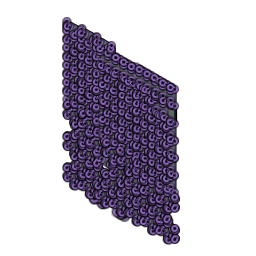
Press Fit v3 (Autodesk Fusion 360 design; units mm, degrees)
Autodesk Fusion 360 part; units mm, degrees
(part 1 of 4)
sketch "Sketch2" plane through (0, 0, 0) normal (0, 0, 1) x (1, 0, 0)
  line L0 (0, 0) -> (50.15, 0)
  line L1 (50.15, 0) -> (50.15, 50.15)
  line L2 (50.15, 50.15) -> (0, 50.15)
  line L3 (0, 50.15) -> (0, 0)
  line L4 (100.15, 0) -> (130.3, 0)
  line L5 (130.3, 0) -> (145.375, 26.1107)
  line L6 (145.375, 26.1107) -> (130.3, 52.2213)
  line L7 (130.3, 52.2213) -> (100.15, 52.2213)
  line L8 (100.15, 52.2213) -> (85.075, 26.1107)
  line L9 (85.075, 26.1107) -> (100.15, 0)
  line L10 (180.3, 50.15) -> (205.45, 50.15)
  line L11 (205.45, 50.15) -> (205.45, 0)
  line L12 (205.45, 0) -> (180.3, 0)
  line L13 (180.3, 0) -> (180.3, 50.15)
  line L14 (23.525, 50.15) -> (26.625, 50.15)
  line L15 (26.625, 50.15) -> (26.625, 40)
  line L16 (26.625, 40) -> (23.525, 40)
  line L17 (23.525, 40) -> (23.525, 50.15)
  line L18 (0, 26.625) -> (10.15, 26.625)
  line L19 (10.15, 26.625) -> (10.15, 23.525)
  line L20 (10.15, 23.525) -> (0, 23.525)
  line L21 (0, 23.525) -> (0, 26.625)
  line L22 (50.15, 26.625) -> (40, 26.625)
  line L23 (40, 26.625) -> (40, 23.525)
  line L24 (40, 23.525) -> (50.15, 23.525)
  line L25 (50.15, 23.525) -> (50.15, 26.625)
  line L26 (26.625, 0) -> (23.525, 0)
  line L27 (23.525, 0) -> (23.525, 10.15)
  line L28 (23.525, 10.15) -> (26.625, 10.15)
  line L29 (26.625, 10.15) -> (26.625, 0)
  line L30 (100.15, 52.2213) -> (130.3, 0) construction
  line L31 (130.3, 52.2213) -> (100.15, 0) construction
  line L32 (85.075, 26.1107) -> (145.375, 26.1107) construction
  line L33 (192.875, 50.15) -> (192.875, 0) construction
  line L34 (25.075, 50.15) -> (25.075, -50.15) construction
  line L35 (0, 25.075) -> (50.15, 25.075) construction
  line L36 (99.2551, 50.6713) -> (101.9398, 52.2213)
  line L37 (101.9398, 52.2213) -> (107.0148, 43.4312)
  line L38 (107.0148, 43.4312) -> (104.3301, 41.8812)
  line L39 (104.3301, 41.8812) -> (99.2551, 50.6713)
  line L40 (128.5102, 52.2213) -> (131.1949, 50.6713)
  line L41 (131.1949, 50.6713) -> (126.1199, 41.8812)
  line L42 (126.1199, 41.8812) -> (123.4352, 43.4312)
  line L43 (123.4352, 43.4312) -> (128.5102, 52.2213)
  line L44 (144.4801, 27.6607) -> (144.4801, 24.5607)
  line L45 (144.4801, 24.5607) -> (134.3301, 24.5607)
  line L46 (134.3301, 24.5607) -> (134.3301, 27.6607)
  line L47 (134.3301, 27.6607) -> (144.4801, 27.6607)
  line L48 (128.5102, 0) -> (131.1949, 1.55)
  line L49 (131.1949, 1.55) -> (126.1199, 10.3402)
  line L50 (126.1199, 10.3402) -> (123.4352, 8.7902)
  line L51 (123.4352, 8.7902) -> (128.5102, 0)
  line L52 (101.9398, 0) -> (99.2551, 1.55)
  line L53 (99.2551, 1.55) -> (104.3301, 10.3402)
  line L54 (104.3301, 10.3402) -> (107.0148, 8.7902)
  line L55 (107.0148, 8.7902) -> (101.9398, 0)
  line L56 (85.9699, 24.5607) -> (85.9699, 27.6607)
  line L57 (85.9699, 27.6607) -> (96.1199, 27.6607)
  line L58 (96.1199, 27.6607) -> (96.1199, 24.5607)
  line L59 (96.1199, 24.5607) -> (85.9699, 24.5607)
  line L60 (191.325, 0) -> (194.425, 0)
  line L61 (194.425, 0) -> (194.425, 10.15)
  line L62 (194.425, 10.15) -> (191.325, 10.15)
  line L63 (191.325, 10.15) -> (191.325, 0)
  line L64 (191.325, 50.15) -> (194.425, 50.15)
  line L65 (194.425, 50.15) -> (194.425, 40)
  line L66 (194.425, 40) -> (191.325, 40)
  line L67 (191.325, 40) -> (191.325, 50.15)
  point P0 (115.225, 26.1107)
  dimension "d5" = 3.1
  dimension "d8" = 10.15
  dimension "d9" = 30.15
  dimension "d10" = 50.15
  dimension "d12" = 25.15
  dimension "d13" = 50.15
  dimension "d14" = 50
  dimension "d15" = 50
  dimension "d20" = 50.15
  constraint horizontal L0
  constraint vertical L1
  constraint horizontal L2
  constraint vertical L3
  constraint coincident L0.start L3.end
  constraint horizontal L4
  constraint horizontal L10
  constraint vertical L11
  constraint horizontal L12
  constraint vertical L13
  constraint horizontal L14
  constraint vertical L15
  constraint horizontal L16
  constraint vertical L17
  constraint coincident L2 L14.start
  constraint horizontal L18
  constraint vertical L19
  constraint horizontal L20
  constraint vertical L21
  constraint horizontal L22
  constraint vertical L23
  constraint horizontal L24
  constraint vertical L25
  constraint coincident L1 L22.start
  constraint vertical L27
  constraint horizontal L28
  constraint vertical L29
  constraint coincident L0 L26.start
  constraint horizontal L32
  constraint midpoint L10 L33.start
  constraint midpoint L12 L33.end
  constraint midpoint L2 L34.start
  constraint midpoint L21 L35.start
  constraint midpoint L25 L35.end
  constraint vertical L34
  constraint horizontal L35
  constraint perpendicular L36 L37
  constraint parallel L36 L38
  constraint parallel L37 L39
  constraint coincident L7 L36.end
  constraint coincident L8 L36.start
  constraint perpendicular L40 L41
  constraint parallel L40 L42
  constraint parallel L41 L43
  constraint coincident L6 L40.end
  constraint coincident L7 L40.start
  constraint perpendicular L44 L45
  constraint parallel L44 L46
  constraint parallel L45 L47
  constraint coincident L5 L44.end
  constraint perpendicular L32 L44
  constraint coincident L6 L44.start
  constraint perpendicular L48 L49
  constraint parallel L48 L50
  constraint parallel L49 L51
  constraint perpendicular L30 L48
  constraint coincident L4 L48.start
  constraint perpendicular L52 L53
  constraint parallel L52 L54
  constraint parallel L53 L55
  constraint coincident L9 L52.end
  constraint coincident L4 L52.start
  constraint perpendicular L56 L57
  constraint parallel L56 L58
  constraint parallel L57 L59
  constraint coincident L8 L56.end
  constraint perpendicular L4 L56
  constraint coincident L9 L56.start
  constraint symmetric L31 L53 L55
  constraint symmetric L30 L37 L39
  constraint symmetric L31 L41 L43
  constraint symmetric L30 L49 L51
  constraint equal L16 L19
  constraint equal L16 L23
  constraint equal L23 L28
  constraint equal L28 L58
  constraint equal L38 L58
  constraint equal L38 L42
  constraint equal L42 L46
  constraint equal L46 L50
  constraint equal L50 L54
  constraint equal L39 L57
  constraint equal L39 L43
  constraint equal L43 L47
  constraint equal L47 L49
  constraint equal L49 L55
  constraint symmetric L0 L2 L35
  constraint equal L15 L59
  constraint equal L15 L20
  constraint equal L20 L24
  constraint equal L24 L29
  constraint collinear L0 L4
  constraint horizontal L60
  constraint vertical L61
  constraint horizontal L62
  constraint vertical L63
  constraint coincident L12 L60.start
  constraint horizontal L64
  constraint vertical L65
  constraint horizontal L66
  constraint vertical L67
  constraint coincident L10 L64.start
  constraint collinear L4 L12
  constraint equal L61 L65
  constraint equal L45 L65
  constraint equal L62 L66
  constraint equal L50 L62
  constraint midpoint L0 L34
  constraint collinear L3 L21
  measures "d5" distance of L18.end L19.end
  measures "d8" distance of L56.end L57.end
  measures "d9" distance of L4.start L4.end
  measures "d10" distance of L0.end L1.end
  measures "d12" distance of L11.end L12.end
  measures "d13" distance of L10.end L11.end
  measures "d14" distance of L0.end L4.start
  measures "d15" distance of L4.end L12.end
  measures "d20" distance of L0.start L0.end
extrude "Extrude1" add sketch "Sketch2" along normal blind 5 contours L0 L1 L2 L3 L15 L16 L17 L18 L19 L20 L22 L23 L24 L27 L28 L29 | L4 L5 L6 L7 L8 L9 L37 L38 L39 L41 L42 L43 L45 L46 L47 L49 L50 L51 L53 L54 L55 L57 L58 L59 | L10 L11 L12 L13 L61 L62 L63 L65 L66 L67 makes body 1 at (11.225, 38.925, 0) makes body 2 at (112.4883, 31.8842, 0) makes body 3 at (183.975, 30.05, 0)
sketch "Sketch7" plane through (0, 0, 0) normal (0, 0, -1) x (1, 0, 0)
  line L0 (50.15, -50.15) -> (50.15, -26.625)
  line L1 (50.15, -26.625) -> (40, -26.625)
  line L2 (40, -26.625) -> (40, -23.525)
  line L3 (40, -23.525) -> (50.15, -23.525)
  line L4 (50.15, -23.525) -> (50.15, 0)
  line L5 (50.15, 0) -> (26.625, 0)
  line L6 (26.625, 0) -> (26.625, -10.15)
  line L7 (26.625, -10.15) -> (23.525, -10.15)
  line L8 (23.525, -10.15) -> (23.525, 0)
  line L9 (23.525, 0) -> (0, 0)
  line L10 (0, 0) -> (0, -23.525)
  line L11 (0, -23.525) -> (10.15, -23.525)
  line L12 (10.15, -23.525) -> (10.15, -26.625)
  line L13 (10.15, -26.625) -> (0, -26.625)
  line L14 (0, -26.625) -> (0, -50.15)
  line L15 (0, -50.15) -> (23.525, -50.15)
  line L16 (23.525, -50.15) -> (23.525, -40)
  line L17 (23.525, -40) -> (26.625, -40)
  line L18 (26.625, -40) -> (26.625, -50.15)
  line L19 (26.625, -50.15) -> (50.15, -50.15)
  line L20 (144.4801, -24.5607) -> (131.1949, -1.55)
  line L21 (131.1949, -1.55) -> (126.1199, -10.3402)
  line L22 (126.1199, -10.3402) -> (123.4352, -8.7902)
  line L23 (123.4352, -8.7902) -> (128.5102, 0)
  line L24 (128.5102, 0) -> (101.9398, 0)
  line L25 (101.9398, 0) -> (107.0148, -8.7902)
  line L26 (107.0148, -8.7902) -> (104.3301, -10.3402)
  line L27 (104.3301, -10.3402) -> (99.2551, -1.55)
  line L28 (99.2551, -1.55) -> (85.9699, -24.5607)
  line L29 (85.9699, -24.5607) -> (96.1199, -24.5607)
  line L30 (96.1199, -24.5607) -> (96.1199, -27.6607)
  line L31 (96.1199, -27.6607) -> (85.9699, -27.6607)
  line L32 (85.9699, -27.6607) -> (99.2551, -50.6713)
  line L33 (99.2551, -50.6713) -> (104.3301, -41.8812)
  line L34 (104.3301, -41.8812) -> (107.0148, -43.4312)
  line L35 (107.0148, -43.4312) -> (101.9398, -52.2213)
  line L36 (101.9398, -52.2213) -> (128.5102, -52.2213)
  line L37 (128.5102, -52.2213) -> (123.4352, -43.4312)
  line L38 (123.4352, -43.4312) -> (126.1199, -41.8812)
  line L39 (126.1199, -41.8812) -> (131.1949, -50.6713)
  line L40 (131.1949, -50.6713) -> (144.4801, -27.6607)
  line L41 (144.4801, -27.6607) -> (134.3301, -27.6607)
  line L42 (134.3301, -27.6607) -> (134.3301, -24.5607)
  line L43 (134.3301, -24.5607) -> (144.4801, -24.5607)
  line L44 (194.425, -40) -> (194.425, -50.15)
  line L45 (194.425, -50.15) -> (205.45, -50.15)
  line L46 (205.45, -50.15) -> (205.45, 0)
  line L47 (205.45, 0) -> (194.425, 0)
  line L48 (194.425, 0) -> (194.425, -10.15)
  line L49 (194.425, -10.15) -> (191.325, -10.15)
  line L50 (191.325, -10.15) -> (191.325, 0)
  line L51 (191.325, 0) -> (180.3, 0)
  line L52 (180.3, 0) -> (180.3, -50.15)
  line L53 (180.3, -50.15) -> (191.325, -50.15)
  line L54 (191.325, -50.15) -> (191.325, -40)
  line L55 (191.325, -40) -> (194.425, -40)
chamfer "Chamfer1" distance 1.5 angle 45 24 edges at (101.9398, 52.2213, 2.5) (85.9699, 27.6607, 2.5) (128.5102, 52.2213, 2.5) (99.2551, 1.55, 2.5) (101.9398, 0, 2.5) (128.5102, 0, 2.5) (131.1949, 1.55, 2.5) (144.4801, 27.6607, 2.5) (131.1949, 50.6713, 2.5) (144.4801, 24.5607, 2.5) (85.9699, 24.5607, 2.5) (99.2551, 50.6713, 2.5) (23.525, 50.15, 2.5) (26.625, 50.15, 2.5) (0, 26.625, 2.5) (0, 23.525, 2.5) (26.625, 0, 2.5) (50.15, 23.525, 2.5) (23.525, 0, 2.5) (50.15, 26.625, 2.5) (191.325, 50.15, 2.5) (194.425, 50.15, 2.5) (194.425, 0, 2.5) (191.325, 0, 2.5) on bodies 1 2 3
sketch "Sketch5" plane through (0, 0, 5) normal (0, 0, 1) x (-1, 0, 0)
  line L0 (-50.15, -28.125) -> (-50.15, -50.15)
  line L1 (-50.15, -50.15) -> (-28.125, -50.15)
  line L2 (-26.625, -48.65) -> (-26.625, -40)
  line L3 (-26.625, -40) -> (-23.525, -40)
  line L4 (-23.525, -40) -> (-23.525, -48.65)
  line L5 (-22.025, -50.15) -> (0, -50.15)
  line L6 (0, -50.15) -> (0, -28.125)
  line L7 (-1.5, -26.625) -> (-10.15, -26.625)
  line L8 (-10.15, -26.625) -> (-10.15, -23.525)
  line L9 (-10.15, -23.525) -> (-1.5, -23.525)
  line L10 (0, -22.025) -> (0, 0)
  line L11 (0, 0) -> (-22.025, 0)
  line L12 (-23.525, -1.5) -> (-23.525, -10.15)
  line L13 (-23.525, -10.15) -> (-26.625, -10.15)
  line L14 (-26.625, -10.15) -> (-26.625, -1.5)
  line L15 (-28.125, 0) -> (-50.15, 0)
  line L16 (-50.15, 0) -> (-50.15, -22.025)
  line L17 (-48.65, -23.525) -> (-40, -23.525)
  line L18 (-40, -23.525) -> (-40, -26.625)
  line L19 (-40, -26.625) -> (-48.65, -26.625)
  line L20 (-131.9449, -2.849) -> (-143.7301, -23.2616)
  line L21 (-142.9801, -24.5607) -> (-134.3301, -24.5607)
  line L22 (-134.3301, -24.5607) -> (-134.3301, -27.6607)
  line L23 (-134.3301, -27.6607) -> (-142.9801, -27.6607)
  line L24 (-143.7301, -28.9597) -> (-131.9449, -49.3723)
  line L25 (-130.4449, -49.3723) -> (-126.1199, -41.8812)
  line L26 (-126.1199, -41.8812) -> (-123.4352, -43.4312)
  line L27 (-123.4352, -43.4312) -> (-127.7602, -50.9223)
  line L28 (-127.0102, -52.2213) -> (-103.4398, -52.2213)
  line L29 (-102.6898, -50.9223) -> (-107.0148, -43.4312)
  line L30 (-107.0148, -43.4312) -> (-104.3301, -41.8812)
  line L31 (-104.3301, -41.8812) -> (-100.0051, -49.3723)
  line L32 (-98.5051, -49.3723) -> (-86.7199, -28.9597)
  line L33 (-87.4699, -27.6607) -> (-96.1199, -27.6607)
  line L34 (-96.1199, -27.6607) -> (-96.1199, -24.5607)
  line L35 (-96.1199, -24.5607) -> (-87.4699, -24.5607)
  line L36 (-86.7199, -23.2616) -> (-98.5051, -2.849)
  line L37 (-100.0051, -2.849) -> (-104.3301, -10.3402)
  line L38 (-104.3301, -10.3402) -> (-107.0148, -8.7902)
  line L39 (-107.0148, -8.7902) -> (-102.6898, -1.299)
  line L40 (-103.4398, 0) -> (-127.0102, 0)
  line L41 (-127.7602, -1.299) -> (-123.4352, -8.7902)
  line L42 (-123.4352, -8.7902) -> (-126.1199, -10.3402)
  line L43 (-126.1199, -10.3402) -> (-130.4449, -2.849)
  line L44 (-194.425, -48.65) -> (-194.425, -40)
  line L45 (-194.425, -40) -> (-191.325, -40)
  line L46 (-191.325, -40) -> (-191.325, -48.65)
  line L47 (-189.825, -50.15) -> (-180.3, -50.15)
  line L48 (-180.3, -50.15) -> (-180.3, 0)
  line L49 (-180.3, 0) -> (-189.825, 0)
  line L50 (-191.325, -1.5) -> (-191.325, -10.15)
  line L51 (-191.325, -10.15) -> (-194.425, -10.15)
  line L52 (-194.425, -10.15) -> (-194.425, -1.5)
  line L53 (-195.925, 0) -> (-205.45, 0)
  line L54 (-205.45, 0) -> (-205.45, -50.15)
  line L55 (-205.45, -50.15) -> (-195.925, -50.15)
  line L56 (-48.65, -26.625) -> (-50.15, -28.125)
  line L57 (-28.125, -50.15) -> (-26.625, -48.65)
  line L58 (-23.525, -48.65) -> (-22.025, -50.15)
  line L59 (0, -28.125) -> (-1.5, -26.625)
  line L60 (-1.5, -23.525) -> (0, -22.025)
  line L61 (-22.025, 0) -> (-23.525, -1.5)
  line L62 (-26.625, -1.5) -> (-28.125, 0)
  line L63 (-50.15, -22.025) -> (-48.65, -23.525)
  line L64 (-100.0051, -49.3723) -> (-98.5051, -49.3723)
  line L65 (-86.7199, -28.9597) -> (-87.4699, -27.6607)
  line L66 (-87.4699, -24.5607) -> (-86.7199, -23.2616)
  line L67 (-98.5051, -2.849) -> (-100.0051, -2.849)
  line L68 (-102.6898, -1.299) -> (-103.4398, 0)
  line L69 (-127.0102, 0) -> (-127.7602, -1.299)
  line L70 (-130.4449, -2.849) -> (-131.9449, -2.849)
  line L71 (-143.7301, -23.2616) -> (-142.9801, -24.5607)
  line L72 (-142.9801, -27.6607) -> (-143.7301, -28.9597)
  line L73 (-131.9449, -49.3723) -> (-130.4449, -49.3723)
  line L74 (-127.7602, -50.9223) -> (-127.0102, -52.2213)
  line L75 (-103.4398, -52.2213) -> (-102.6898, -50.9223)
  line L76 (-189.825, 0) -> (-191.325, -1.5)
  line L77 (-194.425, -1.5) -> (-195.925, 0)
  line L78 (-195.925, -50.15) -> (-194.425, -48.65)
  line L79 (-191.325, -48.65) -> (-189.825, -50.15)
pattern_linear "R-Pattern1" count 5 spacing 75 along (0, 1, 0) count 5 spacing 275 along (1, 0, 0) of bodies 3 2 1 makes body 4 at (11.225, 113.925, 0) makes body 5 at (11.225, 188.925, 0) makes body 6 at (11.225, 263.925, 0) makes body 7 at (11.225, 338.925, 0) makes body 8 at (286.225, 38.925, 0) makes body 9 at (286.225, 113.925, 0) makes body 10 at (286.225, 188.925, 0) makes body 11 at (286.225, 263.925, 0) makes body 12 at (286.225, 338.925, 0) makes body 13 at (561.225, 38.925, 0) makes body 14 at (561.225, 113.925, 0) makes body 15 at (561.225, 188.925, 0) makes body 16 at (561.225, 263.925, 0) makes body 17 at (561.225, 338.925, 0) makes body 18 at (836.225, 38.925, 0) makes body 19 at (836.225, 113.925, 0) makes body 20 at (836.225, 188.925, 0) makes body 21 at (836.225, 263.925, 0) makes body 22 at (836.225, 338.925, 0) makes body 23 at (1111.225, 38.925, 0) makes body 24 at (1111.225, 113.925, 0) makes body 25 at (1111.225, 188.925, 0) makes body 26 at (1111.225, 263.925, 0) makes body 27 at (1111.225, 338.925, 0) makes body 28 at (112.4883, 106.8842, 0) makes body 29 at (112.4883, 181.8842, 0) makes body 30 at (112.4883, 256.8842, 0) makes body 31 at (112.4883, 331.8842, 0) makes body 32 at (387.4883, 31.8842, 0) makes body 33 at (387.4883, 106.8842, 0) makes body 34 at (387.4883, 181.8842, 0) makes body 35 at (387.4883, 256.8842, 0) makes body 36 at (387.4883, 331.8842, 0) makes body 37 at (662.4883, 31.8842, 0) makes body 38 at (662.4883, 106.8842, 0) makes body 39 at (662.4883, 181.8842, 0) makes body 40 at (662.4883, 256.8842, 0) makes body 41 at (662.4883, 331.8842, 0) makes body 42 at (937.4883, 31.8842, 0) makes body 43 at (937.4883, 106.8842, 0) makes body 44 at (937.4883, 181.8842, 0) makes body 45 at (937.4883, 256.8842, 0) makes body 46 at (937.4883, 331.8842, 0) makes body 47 at (1212.4883, 31.8842, 0) makes body 48 at (1212.4883, 106.8842, 0) makes body 49 at (1212.4883, 181.8842, 0) makes body 50 at (1212.4883, 256.8842, 0) makes body 51 at (1212.4883, 331.8842, 0) makes body 52 at (183.975, 105.05, 0) makes body 53 at (201.775, 180.05, 0) makes body 54 at (183.975, 255.05, 0) makes body 55 at (183.975, 330.05, 0) makes body 56 at (458.975, 30.05, 0) makes body 57 at (458.975, 105.05, 0) makes body 58 at (476.775, 180.05, 0) makes body 59 at (458.975, 255.05, 0) makes body 60 at (458.975, 330.05, 0) makes body 61 at (733.975, 30.05, 0) makes body 62 at (733.975, 105.05, 0) makes body 63 at (733.975, 180.05, 0) makes body 64 at (733.975, 255.05, 0) makes body 65 at (733.975, 330.05, 0) makes body 66 at (1008.975, 30.05, 0) makes body 67 at (1008.975, 105.05, 0) makes body 68 at (1008.975, 180.05, 0) makes body 69 at (1008.975, 255.05, 0) makes body 70 at (1008.975, 330.05, 0) makes body 71 at (1283.975, 30.05, 0) makes body 72 at (1283.975, 105.05, 0) makes body 73 at (1283.975, 180.05, 0) makes body 74 at (1283.975, 255.05, 0) makes body 75 at (1283.975, 330.05, 0)
copy_body "Body->Comp1" bodies 1 removing the originals makes body 76 in component "Component"
copy_body "Body->Comp2" bodies 2 removing the originals makes body 77 in component "Component'"
copy_body "Body->Comp3" bodies 3 removing the originals makes body 78 in component "Component''"
copy_body "Body->Comp4" bodies 4 removing the originals makes body 79 in component "Component'''"
copy_body "Body->Comp5" bodies 5 removing the originals makes body 80 in component "Component''''"
copy_body "Body->Comp6" bodies 6 removing the originals makes body 81 in component "Component'''''"
copy_body "Body->Comp7" bodies 7 removing the originals makes body 82 in component "Component''''''"
copy_body "Body->Comp8" bodies 8 removing the originals makes body 83 in component "Component'''''''"
copy_body "Body->Comp9" bodies 9 removing the originals makes body 84 in component "Component''''''''"
copy_body "Body->Comp10" bodies 10 removing the originals makes body 85 in component "Component'''''''''"
copy_body "Body->Comp11" bodies 11 removing the originals makes body 86 in component "Component''''''''''"
copy_body "Body->Comp12" bodies 12 removing the originals makes body 87 in component "Component'''''''''''"
copy_body "Body->Comp13" bodies 13 removing the originals makes body 88 in component "Component''''''''''''"
copy_body "Body->Comp14" bodies 14 removing the originals makes body 89 in component "Component'''''''''''''"
copy_body "Body->Comp15" bodies 15 removing the originals makes body 90 in component "Component''''''''''''''"
copy_body "Body->Comp16" bodies 16 removing the originals makes body 91 in component "Component'''''''''''''''"
copy_body "Body->Comp17" bodies 17 removing the originals makes body 92 in component "Component''''''''''''''''"
copy_body "Body->Comp18" bodies 18 removing the originals makes body 93 in component "Component'''''''''''''''''"
copy_body "Body->Comp19" bodies 19 removing the originals makes body 94 in component "Component''''''''''''''''''"
copy_body "Body->Comp20" bodies 20 removing the originals makes body 95 in component "Component'''''''''''''''''''"
copy_body "Body->Comp21" bodies 21 removing the originals makes body 96 in component "Component''''''''''''''''''''"
copy_body "Body->Comp22" bodies 22 removing the originals makes body 97 in component "Component'''''''''''''''''''''"
copy_body "Body->Comp23" bodies 23 removing the originals makes body 98 in component "Component''''''''''''''''''''''"
copy_body "Body->Comp24" bodies 24 removing the originals makes body 99 in component "Component'''''''''''''''''''''''"
copy_body "Body->Comp25" bodies 25 removing the originals makes body 100 in component "Component''''''''''''''''''''''''"
copy_body "Body->Comp26" bodies 26 removing the originals makes body 101 in component "Component'''''''''''''''''''''''''"
copy_body "Body->Comp27" bodies 27 removing the originals makes body 102 in component "Component''''''''''''''''''''''''''"
copy_body "Body->Comp28" bodies 28 removing the originals makes body 103 in component "Component'''''''''''''''''''''''''''"
copy_body "Body->Comp29" bodies 29 removing the originals makes body 104 in component "Component''''''''''''''''''''''''''''"
copy_body "Body->Comp30" bodies 30 removing the originals makes body 105 in component "Component'''''''''''''''''''''''''''''"
copy_body "Body->Comp31" bodies 31 removing the originals makes body 106 in component "Component''''''''''''''''''''''''''''''"
copy_body "Body->Comp32" bodies 32 removing the originals makes body 107 in component "Component'''''''''''''''''''''''''''''''"
copy_body "Body->Comp33" bodies 33 removing the originals makes body 108 in component "Component''''''''''''''''''''''''''''''''"
copy_body "Body->Comp34" bodies 34 removing the originals makes body 109 in component "Component'''''''''''''''''''''''''''''''''"
copy_body "Body->Comp35" bodies 35 removing the originals makes body 110 in component "Component''''''''''''''''''''''''''''''''''"
copy_body "Body->Comp36" bodies 36 removing the originals makes body 111 in component "Component'''''''''''''''''''''''''''''''''''"
copy_body "Body->Comp37" bodies 37 removing the originals makes body 112 in component "Component''''''''''''''''''''''''''''''''''''"
copy_body "Body->Comp38" bodies 38 removing the originals makes body 113 in component "Component'''''''''''''''''''''''''''''''''''''"
copy_body "Body->Comp39" bodies 39 removing the originals makes body 114 in component "Component''''''''''''''''''''''''''''''''''''''"
copy_body "Body->Comp40" bodies 40 removing the originals makes body 115 in component "Component'''''''''''''''''''''''''''''''''''''''"
copy_body "Body->Comp41" bodies 41 removing the originals makes body 116 in component "Component''''''''''''''''''''''''''''''''''''''''"
copy_body "Body->Comp42" bodies 42 removing the originals makes body 117 in component "Component'''''''''''''''''''''''''''''''''''''''''"
copy_body "Body->Comp43" bodies 43 removing the originals makes body 118 in component "Component''''''''''''''''''''''''''''''''''''''''''"
copy_body "Body->Comp44" bodies 44 removing the originals makes body 119 in component "Component'''''''''''''''''''''''''''''''''''''''''''"
copy_body "Body->Comp45" bodies 45 removing the originals makes body 120 in component "Component''''''''''''''''''''''''''''''''''''''''''''"
copy_body "Body->Comp46" bodies 46 removing the originals makes body 121 in component "Component'''''''''''''''''''''''''''''''''''''''''''''"
copy_body "Body->Comp47" bodies 47 removing the originals makes body 122 in component "Component''''''''''''''''''''''''''''''''''''''''''''''"
copy_body "Body->Comp48" bodies 48 removing the originals makes body 123 in component "Component'''''''''''''''''''''''''''''''''''''''''''''''"
copy_body "Body->Comp49" bodies 49 removing the originals makes body 124 in component "Component''''''''''''''''''''''''''''''''''''''''''''''''"
copy_body "Body->Comp50" bodies 50 removing the originals makes body 125 in component "Component'''''''''''''''''''''''''''''''''''''''''''''''''"
copy_body "Body->Comp51" bodies 51 removing the originals makes body 126 in component "Component''''''''''''''''''''''''''''''''''''''''''''''''''"
copy_body "Body->Comp52" bodies 52 removing the originals makes body 127 in component "Component'''''''''''''''''''''''''''''''''''''''''''''''''''"
copy_body "Body->Comp53" bodies 53 removing the originals makes body 128 in component "Component''''''''''''''''''''''''''''''''''''''''''''''''''''"
copy_body "Body->Comp54" bodies 54 removing the originals makes body 129 in component "Component'''''''''''''''''''''''''''''''''''''''''''''''''''''"
copy_body "Body->Comp55" bodies 55 removing the originals makes body 130 in component "Component''''''''''''''''''''''''''''''''''''''''''''''''''''''"
copy_body "Body->Comp56" bodies 56 removing the originals makes body 131 in component "Component'''''''''''''''''''''''''''''''''''''''''''''''''''''''"
copy_body "Body->Comp57" bodies 57 removing the originals makes body 132 in component "Component''''''''''''''''''''''''''''''''''''''''''''''''''''''''"
copy_body "Body->Comp58" bodies 58 removing the originals makes body 133 in component "Component'''''''''''''''''''''''''''''''''''''''''''''''''''''''''"
copy_body "Body->Comp59" bodies 59 removing the originals makes body 134 in component "Component''''''''''''''''''''''''''''''''''''''''''''''''''''''''''"
copy_body "Body->Comp60" bodies 60 removing the originals makes body 135 in component "Component'''''''''''''''''''''''''''''''''''''''''''''''''''''''''''"
copy_body "Body->Comp61" bodies 61 removing the originals makes body 136 in component "Component''''''''''''''''''''''''''''''''''''''''''''''''''''''''''''"
copy_body "Body->Comp62" bodies 62 removing the originals makes body 137 in component "Component'''''''''''''''''''''''''''''''''''''''''''''''''''''''''''''"
copy_body "Body->Comp63" bodies 63 removing the originals makes body 138 in component "Component''''''''''''''''''''''''''''''''''''''''''''''''''''''''''''''"
copy_body "Body->Comp64" bodies 64 removing the originals makes body 139 in component "Component'''''''''''''''''''''''''''''''''''''''''''''''''''''''''''''''"
copy_body "Body->Comp65" bodies 65 removing the originals makes body 140 in component "Component''''''''''''''''''''''''''''''''''''''''''''''''''''''''''''''''"
copy_body "Body->Comp66" bodies 66 removing the originals makes body 141 in component "Component'''''''''''''''''''''''''''''''''''''''''''''''''''''''''''''''''"
copy_body "Body->Comp67" bodies 67 removing the originals makes body 142 in component "Component''''''''''''''''''''''''''''''''''''''''''''''''''''''''''''''''''"
copy_body "Body->Comp68" bodies 68 removing the originals makes body 143 in component "Component'''''''''''''''''''''''''''''''''''''''''''''''''''''''''''''''''''"
copy_body "Body->Comp69" bodies 69 removing the originals makes body 144 in component "Component''''''''''''''''''''''''''''''''''''''''''''''''''''''''''''''''''''"
copy_body "Body->Comp70" bodies 70 removing the originals makes body 145 in component "Component'''''''''''''''''''''''''''''''''''''''''''''''''''''''''''''''''''''"
copy_body "Body->Comp71" bodies 71 removing the originals makes body 146 in component "Component''''''''''''''''''''''''''''''''''''''''''''''''''''''''''''''''''''''"
copy_body "Body->Comp72" bodies 72 removing the originals makes body 147 in component "Component'''''''''''''''''''''''''''''''''''''''''''''''''''''''''''''''''''''''"
copy_body "Body->Comp73" bodies 73 removing the originals makes body 148 in component "Component''''''''''''''''''''''''''''''''''''''''''''''''''''''''''''''''''''''''"
copy_body "Body->Comp74" bodies 74 removing the originals makes body 149 in component "Component'''''''''''''''''''''''''''''''''''''''''''''''''''''''''''''''''''''''''"
copy_body "Body->Comp75" bodies 75 removing the originals makes body 150 in component "Component''''''''''''''''''''''''''''''''''''''''''''''''''''''''''''''''''''''''''"
other "Arrange1"
sketch "Sketch6" plane through (-20.8162, 0, 446.9337) normal (0, -1, 0) x (0, 0, -1)
  line L0 (70.2593, 390.3874) -> (78.9093, 390.3874)
  line L1 (80.4093, 391.8874) -> (80.4093, 401.4124)
  line L2 (80.4093, 401.4124) -> (30.2593, 401.4124)
  line L3 (30.2593, 401.4124) -> (30.2593, 391.8874)
  line L4 (31.7593, 390.3874) -> (40.4093, 390.3874)
  line L5 (40.4093, 390.3874) -> (40.4093, 387.2874)
  line L6 (40.4093, 387.2874) -> (31.7593, 387.2874)
  line L7 (30.2593, 385.7874) -> (30.2593, 376.2624)
  line L8 (30.2593, 376.2624) -> (80.4093, 376.2624)
  line L9 (80.4093, 376.2624) -> (80.4093, 385.7874)
  line L10 (78.9093, 387.2874) -> (70.2593, 387.2874)
  line L11 (70.2593, 387.2874) -> (70.2593, 390.3874)
  line L12 (179.8991, 152.4871) -> (188.5491, 152.4871)
  line L13 (190.0491, 153.9871) -> (190.0491, 163.5121)
  line L14 (190.0491, 163.5121) -> (139.8991, 163.5121)
  line L15 (139.8991, 163.5121) -> (139.8991, 153.9871)
  line L16 (141.3991, 152.4871) -> (150.0491, 152.4871)
  line L17 (150.0491, 152.4871) -> (150.0491, 149.3871)
  line L18 (150.0491, 149.3871) -> (141.3991, 149.3871)
  line L19 (139.8991, 147.8871) -> (139.8991, 138.3621)
  line L20 (139.8991, 138.3621) -> (190.0491, 138.3621)
  line L21 (190.0491, 138.3621) -> (190.0491, 147.8871)
  line L22 (188.5491, 149.3871) -> (179.8991, 149.3871)
  line L23 (179.8991, 149.3871) -> (179.8991, 152.4871)
  line L24 (23.3078, 252.8413) -> (31.9578, 252.8413)
  line L25 (33.4578, 254.3413) -> (33.4578, 263.8663)
  line L26 (33.4578, 263.8663) -> (-16.6922, 263.8663)
  line L27 (-16.6922, 263.8663) -> (-16.6922, 254.3413)
  line L28 (-15.1922, 252.8413) -> (-6.5422, 252.8413)
  line L29 (-6.5422, 252.8413) -> (-6.5422, 249.7413)
  line L30 (-6.5422, 249.7413) -> (-15.1922, 249.7413)
  line L31 (-16.6922, 248.2413) -> (-16.6922, 238.7163)
  line L32 (-16.6922, 238.7163) -> (33.4578, 238.7163)
  line L33 (33.4578, 238.7163) -> (33.4578, 248.2413)
  line L34 (31.9578, 249.7413) -> (23.3078, 249.7413)
  line L35 (23.3078, 249.7413) -> (23.3078, 252.8413)
  line L36 (23.4138, 171.3912) -> (32.0638, 171.3912)
  line L37 (33.5638, 172.8912) -> (33.5638, 182.4162)
  line L38 (33.5638, 182.4162) -> (-16.5862, 182.4162)
  line L39 (-16.5862, 182.4162) -> (-16.5862, 172.8912)
  line L40 (-15.0862, 171.3912) -> (-6.4362, 171.3912)
  line L41 (-6.4362, 171.3912) -> (-6.4362, 168.2912)
  line L42 (-6.4362, 168.2912) -> (-15.0862, 168.2912)
  line L43 (-16.5862, 166.7912) -> (-16.5862, 157.2662)
  line L44 (-16.5862, 157.2662) -> (33.5638, 157.2662)
  line L45 (33.5638, 157.2662) -> (33.5638, 166.7912)
  line L46 (32.0638, 168.2912) -> (23.4138, 168.2912)
  line L47 (23.4138, 168.2912) -> (23.4138, 171.3912)
  line L48 (278.8594, 388.237) -> (287.5094, 388.237)
  line L49 (289.0094, 389.737) -> (289.0094, 399.262)
  line L50 (289.0094, 399.262) -> (238.8594, 399.262)
  line L51 (238.8594, 399.262) -> (238.8594, 389.737)
  line L52 (240.3594, 388.237) -> (249.0094, 388.237)
  line L53 (249.0094, 388.237) -> (249.0094, 385.137)
  line L54 (249.0094, 385.137) -> (240.3594, 385.137)
  line L55 (238.8594, 383.637) -> (238.8594, 374.112)
  line L56 (238.8594, 374.112) -> (289.0094, 374.112)
  line L57 (289.0094, 374.112) -> (289.0094, 383.637)
  line L58 (287.5094, 385.137) -> (278.8594, 385.137)
  line L59 (278.8594, 385.137) -> (278.8594, 388.237)
  line L60 (226.7094, 388.2371) -> (235.3594, 388.2371)
  line L61 (236.8594, 389.7371) -> (236.8594, 399.2621)
  line L62 (236.8594, 399.2621) -> (186.7094, 399.2621)
  line L63 (186.7094, 399.2621) -> (186.7094, 389.7371)
  line L64 (188.2094, 388.2371) -> (196.8594, 388.2371)
  line L65 (196.8594, 388.2371) -> (196.8594, 385.1371)
  line L66 (196.8594, 385.1371) -> (188.2094, 385.1371)
  line L67 (186.7094, 383.6371) -> (186.7094, 374.1121)
  line L68 (186.7094, 374.1121) -> (236.8594, 374.1121)
  line L69 (236.8594, 374.1121) -> (236.8594, 383.6371)
  line L70 (235.3594, 385.1371) -> (226.7094, 385.1371)
  line L71 (226.7094, 385.1371) -> (226.7094, 388.2371)
  line L72 (-32.676, 117.9662) -> (-32.676, 126.6162)
  line L73 (-34.176, 128.1162) -> (-43.701, 128.1162)
  line L74 (-43.701, 128.1162) -> (-43.701, 77.9662)
  line L75 (-43.701, 77.9662) -> (-34.176, 77.9662)
  line L76 (-32.676, 79.4662) -> (-32.676, 88.1162)
  line L77 (-32.676, 88.1162) -> (-29.576, 88.1162)
  line L78 (-29.576, 88.1162) -> (-29.576, 79.4662)
  line L79 (-28.076, 77.9662) -> (-18.551, 77.9662)
  line L80 (-18.551, 77.9662) -> (-18.551, 128.1162)
  line L81 (-18.551, 128.1162) -> (-28.076, 128.1162)
  line L82 (-29.576, 126.6162) -> (-29.576, 117.9662)
  line L83 (-29.576, 117.9662) -> (-32.676, 117.9662)
  line L84 (-29.6151, 140.2662) -> (-29.6151, 131.6162)
  line L85 (-28.1151, 130.1162) -> (-18.5901, 130.1162)
  line L86 (-18.5901, 130.1162) -> (-18.5901, 180.2662)
  line L87 (-18.5901, 180.2662) -> (-28.1151, 180.2662)
  line L88 (-29.6151, 178.7662) -> (-29.6151, 170.1162)
  line L89 (-29.6151, 170.1162) -> (-32.7151, 170.1162)
  line L90 (-32.7151, 170.1162) -> (-32.7151, 178.7662)
  line L91 (-34.2151, 180.2662) -> (-43.7401, 180.2662)
  line L92 (-43.7401, 180.2662) -> (-43.7401, 130.1162)
  line L93 (-43.7401, 130.1162) -> (-34.2151, 130.1162)
  line L94 (-32.7151, 131.6162) -> (-32.7151, 140.2662)
  line L95 (-32.7151, 140.2662) -> (-29.6151, 140.2662)
  line L96 (-27.6298, 65.8162) -> (-27.6298, 74.4662)
  line L97 (-29.1298, 75.9662) -> (-38.6548, 75.9662)
  line L98 (-38.6548, 75.9662) -> (-38.6548, 25.8162)
  line L99 (-38.6548, 25.8162) -> (-29.1298, 25.8162)
  line L100 (-27.6298, 27.3162) -> (-27.6298, 35.9662)
  line L101 (-27.6298, 35.9662) -> (-24.5298, 35.9662)
  line L102 (-24.5298, 35.9662) -> (-24.5298, 27.3162)
  line L103 (-23.0298, 25.8162) -> (-13.5048, 25.8162)
  line L104 (-13.5048, 25.8162) -> (-13.5048, 75.9662)
  line L105 (-13.5048, 75.9662) -> (-23.0298, 75.9662)
  line L106 (-24.5298, 74.4662) -> (-24.5298, 65.8162)
  line L107 (-24.5298, 65.8162) -> (-27.6298, 65.8162)
  line L108 (75.5991, 152.4873) -> (84.2491, 152.4873)
  line L109 (85.7491, 153.9873) -> (85.7491, 163.5123)
  line L110 (85.7491, 163.5123) -> (35.5991, 163.5123)
  line L111 (35.5991, 163.5123) -> (35.5991, 153.9873)
  line L112 (37.0991, 152.4873) -> (45.7491, 152.4873)
  line L113 (45.7491, 152.4873) -> (45.7491, 149.3873)
  line L114 (45.7491, 149.3873) -> (37.0991, 149.3873)
  line L115 (35.5991, 147.8873) -> (35.5991, 138.3623)
  line L116 (35.5991, 138.3623) -> (85.7491, 138.3623)
  line L117 (85.7491, 138.3623) -> (85.7491, 147.8873)
  line L118 (84.2491, 149.3873) -> (75.5991, 149.3873)
  line L119 (75.5991, 149.3873) -> (75.5991, 152.4873)
  line L120 (18.1092, 307.1412) -> (26.7592, 307.1412)
  line L121 (28.2592, 308.6412) -> (28.2592, 318.1662)
  line L122 (28.2592, 318.1662) -> (-21.8908, 318.1662)
  line L123 (-21.8908, 318.1662) -> (-21.8908, 308.6412)
  line L124 (-20.3908, 307.1412) -> (-11.7408, 307.1412)
  line L125 (-11.7408, 307.1412) -> (-11.7408, 304.0412)
  line L126 (-11.7408, 304.0412) -> (-20.3908, 304.0412)
  line L127 (-21.8908, 302.5412) -> (-21.8908, 293.0162)
  line L128 (-21.8908, 293.0162) -> (28.2592, 293.0162)
  line L129 (28.2592, 293.0162) -> (28.2592, 302.5412)
  line L130 (26.7592, 304.0412) -> (18.1092, 304.0412)
  line L131 (18.1092, 304.0412) -> (18.1092, 307.1412)
  line L132 (314.0876, 176.3303) -> (314.0876, 184.9803)
  line L133 (312.5876, 186.4803) -> (303.0626, 186.4803)
  line L134 (303.0626, 186.4803) -> (303.0626, 136.3303)
  line L135 (303.0626, 136.3303) -> (312.5876, 136.3303)
  line L136 (314.0876, 137.8303) -> (314.0876, 146.4803)
  line L137 (314.0876, 146.4803) -> (317.1876, 146.4803)
  line L138 (317.1876, 146.4803) -> (317.1876, 137.8303)
  line L139 (318.6876, 136.3303) -> (328.2126, 136.3303)
  line L140 (328.2126, 136.3303) -> (328.2126, 186.4803)
  line L141 (328.2126, 186.4803) -> (318.6876, 186.4803)
  line L142 (317.1876, 184.9803) -> (317.1876, 176.3303)
  line L143 (317.1876, 176.3303) -> (314.0876, 176.3303)
  line L144 (70.2592, 336.0874) -> (78.9092, 336.0874)
  line L145 (80.4092, 337.5874) -> (80.4092, 347.1124)
  line L146 (80.4092, 347.1124) -> (30.2592, 347.1124)
  line L147 (30.2592, 347.1124) -> (30.2592, 337.5874)
  line L148 (31.7592, 336.0874) -> (40.4092, 336.0874)
  line L149 (40.4092, 336.0874) -> (40.4092, 332.9874)
  line L150 (40.4092, 332.9874) -> (31.7592, 332.9874)
  line L151 (30.2592, 331.4874) -> (30.2592, 321.9624)
  line L152 (30.2592, 321.9624) -> (80.4092, 321.9624)
  line L153 (80.4092, 321.9624) -> (80.4092, 331.4874)
  line L154 (78.9092, 332.9874) -> (70.2592, 332.9874)
  line L155 (70.2592, 332.9874) -> (70.2592, 336.0874)
  line L156 (23.3785, 198.5412) -> (32.0285, 198.5412)
  line L157 (33.5285, 200.0412) -> (33.5285, 209.5662)
  line L158 (33.5285, 209.5662) -> (-16.6215, 209.5662)
  line L159 (-16.6215, 209.5662) -> (-16.6215, 200.0412)
  line L160 (-15.1215, 198.5412) -> (-6.4715, 198.5412)
  line L161 (-6.4715, 198.5412) -> (-6.4715, 195.4412)
  line L162 (-6.4715, 195.4412) -> (-15.1215, 195.4412)
  line L163 (-16.6215, 193.9412) -> (-16.6215, 184.4162)
  line L164 (-16.6215, 184.4162) -> (33.5285, 184.4162)
  line L165 (33.5285, 184.4162) -> (33.5285, 193.9412)
  line L166 (32.0285, 195.4412) -> (23.3785, 195.4412)
  line L167 (23.3785, 195.4412) -> (23.3785, 198.5412)
  line L168 (23.3432, 225.6912) -> (31.9932, 225.6912)
  line L169 (33.4932, 227.1912) -> (33.4932, 236.7162)
  line L170 (33.4932, 236.7162) -> (-16.6568, 236.7162)
  line L171 (-16.6568, 236.7162) -> (-16.6568, 227.1912)
  line L172 (-15.1568, 225.6912) -> (-6.5068, 225.6912)
  line L173 (-6.5068, 225.6912) -> (-6.5068, 222.5912)
  line L174 (-6.5068, 222.5912) -> (-15.1568, 222.5912)
  line L175 (-16.6568, 221.0912) -> (-16.6568, 211.5662)
  line L176 (-16.6568, 211.5662) -> (33.4932, 211.5662)
  line L177 (33.4932, 211.5662) -> (33.4932, 221.0912)
  line L178 (31.9932, 222.5912) -> (23.3432, 222.5912)
  line L179 (23.3432, 222.5912) -> (23.3432, 225.6912)
  line L180 (18.1092, 388.591) -> (26.7592, 388.591)
  line L181 (28.2592, 390.091) -> (28.2592, 399.616)
  line L182 (28.2592, 399.616) -> (-21.8908, 399.616)
  line L183 (-21.8908, 399.616) -> (-21.8908, 390.091)
  line L184 (-20.3908, 388.591) -> (-11.7408, 388.591)
  line L185 (-11.7408, 388.591) -> (-11.7408, 385.491)
  line L186 (-11.7408, 385.491) -> (-20.3908, 385.491)
  line L187 (-21.8908, 383.991) -> (-21.8908, 374.466)
  line L188 (-21.8908, 374.466) -> (28.2592, 374.466)
  line L189 (28.2592, 374.466) -> (28.2592, 383.991)
  line L190 (26.7592, 385.491) -> (18.1092, 385.491)
  line L191 (18.1092, 385.491) -> (18.1092, 388.591)
  line L192 (127.7491, 152.4871) -> (136.3991, 152.4871)
  line L193 (137.8991, 153.9871) -> (137.8991, 163.5121)
  line L194 (137.8991, 163.5121) -> (87.7491, 163.5121)
  line L195 (87.7491, 163.5121) -> (87.7491, 153.9871)
  line L196 (89.2491, 152.4871) -> (97.8991, 152.4871)
  line L197 (97.8991, 152.4871) -> (97.8991, 149.3871)
  line L198 (97.8991, 149.3871) -> (89.2491, 149.3871)
  line L199 (87.7491, 147.8871) -> (87.7491, 138.3621)
  line L200 (87.7491, 138.3621) -> (137.8991, 138.3621)
  line L201 (137.8991, 138.3621) -> (137.8991, 147.8871)
  line L202 (136.3991, 149.3871) -> (127.7491, 149.3871)
  line L203 (127.7491, 149.3871) -> (127.7491, 152.4871)
  line L204 (232.0491, 152.487) -> (240.6991, 152.487)
  line L205 (242.1991, 153.987) -> (242.1991, 163.512)
  line L206 (242.1991, 163.512) -> (192.0491, 163.512)
  line L207 (192.0491, 163.512) -> (192.0491, 153.987)
  line L208 (193.5491, 152.487) -> (202.1991, 152.487)
  line L209 (202.1991, 152.487) -> (202.1991, 149.387)
  line L210 (202.1991, 149.387) -> (193.5491, 149.387)
  line L211 (192.0491, 147.887) -> (192.0491, 138.362)
  line L212 (192.0491, 138.362) -> (242.1991, 138.362)
  line L213 (242.1991, 138.362) -> (242.1991, 147.887)
  line L214 (240.6991, 149.387) -> (232.0491, 149.387)
  line L215 (232.0491, 149.387) -> (232.0491, 152.487)
  line L216 (23.449, 144.2412) -> (32.099, 144.2412)
  line L217 (33.599, 145.7412) -> (33.599, 155.2662)
  line L218 (33.599, 155.2662) -> (-16.551, 155.2662)
  line L219 (-16.551, 155.2662) -> (-16.551, 145.7412)
  line L220 (-15.051, 144.2412) -> (-6.401, 144.2412)
  line L221 (-6.401, 144.2412) -> (-6.401, 141.1412)
  line L222 (-6.401, 141.1412) -> (-15.051, 141.1412)
  line L223 (-16.551, 139.6412) -> (-16.551, 130.1162)
  line L224 (-16.551, 130.1162) -> (33.599, 130.1162)
  line L225 (33.599, 130.1162) -> (33.599, 139.6412)
  line L226 (32.099, 141.1412) -> (23.449, 141.1412)
  line L227 (23.449, 141.1412) -> (23.449, 144.2412)
  line L228 (18.1092, 279.9913) -> (26.7592, 279.9913)
  line L229 (28.2592, 281.4913) -> (28.2592, 291.0163)
  line L230 (28.2592, 291.0163) -> (-21.8908, 291.0163)
  line L231 (-21.8908, 291.0163) -> (-21.8908, 281.4913)
  line L232 (-20.3908, 279.9913) -> (-11.7408, 279.9913)
  line L233 (-11.7408, 279.9913) -> (-11.7408, 276.8913)
  line L234 (-11.7408, 276.8913) -> (-20.3908, 276.8913)
  line L235 (-21.8908, 275.3913) -> (-21.8908, 265.8663)
  line L236 (-21.8908, 265.8663) -> (28.2592, 265.8663)
  line L237 (28.2592, 265.8663) -> (28.2592, 275.3913)
  line L238 (26.7592, 276.8913) -> (18.1092, 276.8913)
  line L239 (18.1092, 276.8913) -> (18.1092, 279.9913)
  line L240 (-11.7408, 331.1911) -> (-20.3908, 331.1911)
  line L241 (-21.8908, 329.6911) -> (-21.8908, 320.1661)
  line L242 (-21.8908, 320.1661) -> (28.2592, 320.1661)
  line L243 (28.2592, 320.1661) -> (28.2592, 329.6911)
  line L244 (26.7592, 331.1911) -> (18.1092, 331.1911)
  line L245 (18.1092, 331.1911) -> (18.1092, 334.2911)
  line L246 (18.1092, 334.2911) -> (26.7592, 334.2911)
  line L247 (28.2592, 335.7911) -> (28.2592, 345.3161)
  line L248 (28.2592, 345.3161) -> (-21.8908, 345.3161)
  line L249 (-21.8908, 345.3161) -> (-21.8908, 335.7911)
  line L250 (-20.3908, 334.2911) -> (-11.7408, 334.2911)
  line L251 (-11.7408, 334.2911) -> (-11.7408, 331.1911)
  line L252 (122.4094, 388.2373) -> (131.0594, 388.2373)
  line L253 (132.5594, 389.7373) -> (132.5594, 399.2623)
  line L254 (132.5594, 399.2623) -> (82.4094, 399.2623)
  line L255 (82.4094, 399.2623) -> (82.4094, 389.7373)
  line L256 (83.9094, 388.2373) -> (92.5594, 388.2373)
  line L257 (92.5594, 388.2373) -> (92.5594, 385.1373)
  line L258 (92.5594, 385.1373) -> (83.9094, 385.1373)
  line L259 (82.4094, 383.6373) -> (82.4094, 374.1123)
  line L260 (82.4094, 374.1123) -> (132.5594, 374.1123)
  line L261 (132.5594, 374.1123) -> (132.5594, 383.6373)
  line L262 (131.0594, 385.1373) -> (122.4094, 385.1373)
  line L263 (122.4094, 385.1373) -> (122.4094, 388.2373)
  line L264 (384.9234, 374.4058) -> (396.7086, 353.9932)
  line L265 (398.2086, 353.9932) -> (402.5336, 361.4843)
  line L266 (402.5336, 361.4843) -> (405.2183, 359.9343)
  line L267 (405.2183, 359.9343) -> (400.8933, 352.4432)
  line L268 (401.6433, 351.1442) -> (425.2137, 351.1442)
  line L269 (425.9637, 352.4432) -> (421.6387, 359.9343)
  line L270 (421.6387, 359.9343) -> (424.3234, 361.4843)
  line L271 (424.3234, 361.4843) -> (428.6484, 353.9932)
  line L272 (430.1484, 353.9932) -> (441.9336, 374.4058)
  line L273 (441.1836, 375.7048) -> (432.5336, 375.7048)
  line L274 (432.5336, 375.7048) -> (432.5336, 378.8048)
  line L275 (432.5336, 378.8048) -> (441.1836, 378.8048)
  line L276 (441.9336, 380.1039) -> (430.1484, 400.5165)
  line L277 (428.6484, 400.5165) -> (424.3234, 393.0253)
  line L278 (424.3234, 393.0253) -> (421.6387, 394.5753)
  line L279 (421.6387, 394.5753) -> (425.9637, 402.0665)
  line L280 (425.2137, 403.3655) -> (401.6433, 403.3655)
  line L281 (400.8933, 402.0665) -> (405.2183, 394.5753)
  line L282 (405.2183, 394.5753) -> (402.5336, 393.0253)
  line L283 (402.5336, 393.0253) -> (398.2086, 400.5165)
  line L284 (396.7086, 400.5165) -> (384.9234, 380.1039)
  line L285 (385.6734, 378.8048) -> (394.3234, 378.8048)
  line L286 (394.3234, 378.8048) -> (394.3234, 375.7048)
  line L287 (394.3234, 375.7048) -> (385.6734, 375.7048)
  line L288 (291.0093, 211.7419) -> (302.7946, 191.3293)
  line L289 (304.2946, 191.3293) -> (308.6196, 198.8204)
  line L290 (308.6196, 198.8204) -> (311.3042, 197.2704)
  line L291 (311.3042, 197.2704) -> (306.9792, 189.7793)
  line L292 (307.7292, 188.4803) -> (331.2997, 188.4803)
  line L293 (332.0497, 189.7793) -> (327.7247, 197.2704)
  line L294 (327.7247, 197.2704) -> (330.4093, 198.8204)
  line L295 (330.4093, 198.8204) -> (334.7343, 191.3293)
  line L296 (336.2343, 191.3293) -> (348.0196, 211.7419)
  line L297 (347.2696, 213.0409) -> (338.6196, 213.0409)
  line L298 (338.6196, 213.0409) -> (338.6196, 216.1409)
  line L299 (338.6196, 216.1409) -> (347.2696, 216.1409)
  line L300 (348.0196, 217.44) -> (336.2343, 237.8526)
  line L301 (334.7343, 237.8526) -> (330.4093, 230.3615)
  line L302 (330.4093, 230.3615) -> (327.7247, 231.9115)
  line L303 (327.7247, 231.9115) -> (332.0497, 239.4026)
  line L304 (331.2997, 240.7016) -> (307.7292, 240.7016)
  line L305 (306.9792, 239.4026) -> (311.3042, 231.9115)
  line L306 (311.3042, 231.9115) -> (308.6196, 230.3615)
  line L307 (308.6196, 230.3615) -> (304.2946, 237.8526)
  line L308 (302.7946, 237.8526) -> (291.0093, 217.44)
  line L309 (291.7593, 216.1409) -> (300.4093, 216.1409)
  line L310 (300.4093, 216.1409) -> (300.4093, 213.0409)
  line L311 (300.4093, 213.0409) -> (291.7593, 213.0409)
  line L312 (254.1055, 54.7759) -> (242.3203, 75.1885)
  line L313 (240.8203, 75.1885) -> (236.4953, 67.6973)
  line L314 (236.4953, 67.6973) -> (233.8106, 69.2473)
  line L315 (233.8106, 69.2473) -> (238.1356, 76.7385)
  line L316 (237.3856, 78.0375) -> (213.8152, 78.0375)
  line L317 (213.0652, 76.7385) -> (217.3902, 69.2473)
  line L318 (217.3902, 69.2473) -> (214.7055, 67.6973)
  line L319 (214.7055, 67.6973) -> (210.3805, 75.1885)
  line L320 (208.8805, 75.1885) -> (197.0953, 54.7759)
  line L321 (197.8453, 53.4768) -> (206.4953, 53.4768)
  line L322 (206.4953, 53.4768) -> (206.4953, 50.3768)
  line L323 (206.4953, 50.3768) -> (197.8453, 50.3768)
  line L324 (197.0953, 49.0778) -> (208.8805, 28.6652)
  line L325 (210.3805, 28.6652) -> (214.7055, 36.1563)
  line L326 (214.7055, 36.1563) -> (217.3902, 34.6063)
  line L327 (217.3902, 34.6063) -> (213.0652, 27.1152)
  line L328 (213.8152, 25.8162) -> (237.3856, 25.8162)
  line L329 (238.1356, 27.1152) -> (233.8106, 34.6063)
  line L330 (233.8106, 34.6063) -> (236.4953, 36.1563)
  line L331 (236.4953, 36.1563) -> (240.8203, 28.6652)
  line L332 (242.3203, 28.6652) -> (254.1055, 49.0778)
  line L333 (253.3555, 50.3768) -> (244.7055, 50.3768)
  line L334 (244.7055, 50.3768) -> (244.7055, 53.4768)
  line L335 (244.7055, 53.4768) -> (253.3555, 53.4768)
  line L336 (337.9664, 347.295) -> (349.7516, 326.8824)
  line L337 (351.2516, 326.8824) -> (355.5766, 334.3735)
  line L338 (355.5766, 334.3735) -> (358.2613, 332.8235)
  line L339 (358.2613, 332.8235) -> (353.9363, 325.3324)
  line L340 (354.6863, 324.0333) -> (378.2567, 324.0333)
  line L341 (379.0067, 325.3324) -> (374.6817, 332.8235)
  line L342 (374.6817, 332.8235) -> (377.3664, 334.3735)
  line L343 (377.3664, 334.3735) -> (381.6914, 326.8824)
  line L344 (383.1914, 326.8824) -> (394.9766, 347.295)
  line L345 (394.2266, 348.594) -> (385.5766, 348.594)
  line L346 (385.5766, 348.594) -> (385.5766, 351.694)
  line L347 (385.5766, 351.694) -> (394.2266, 351.694)
  line L348 (394.9766, 352.993) -> (383.1914, 373.4056)
  line L349 (381.6914, 373.4056) -> (377.3664, 365.9145)
  line L350 (377.3664, 365.9145) -> (374.6817, 367.4645)
  line L351 (374.6817, 367.4645) -> (379.0067, 374.9556)
  line L352 (378.2567, 376.2547) -> (354.6863, 376.2547)
  line L353 (353.9363, 374.9556) -> (358.2613, 367.4645)
  line L354 (358.2613, 367.4645) -> (355.5766, 365.9145)
  line L355 (355.5766, 365.9145) -> (351.2516, 373.4056)
  line L356 (349.7516, 373.4056) -> (337.9664, 352.993)
  line L357 (338.7164, 351.694) -> (347.3664, 351.694)
  line L358 (347.3664, 351.694) -> (347.3664, 348.594)
  line L359 (347.3664, 348.594) -> (338.7164, 348.594)
  line L360 (337.9664, 293.0738) -> (349.7516, 272.6613)
  line L361 (351.2516, 272.6613) -> (355.5766, 280.1524)
  line L362 (355.5766, 280.1524) -> (358.2613, 278.6024)
  line L363 (358.2613, 278.6024) -> (353.9363, 271.1113)
  line L364 (354.6863, 269.8122) -> (378.2567, 269.8122)
  line L365 (379.0067, 271.1113) -> (374.6817, 278.6024)
  line L366 (374.6817, 278.6024) -> (377.3664, 280.1524)
  line L367 (377.3664, 280.1524) -> (381.6914, 272.6613)
  line L368 (383.1914, 272.6613) -> (394.9766, 293.0738)
  line L369 (394.2266, 294.3729) -> (385.5766, 294.3729)
  line L370 (385.5766, 294.3729) -> (385.5766, 297.4729)
  line L371 (385.5766, 297.4729) -> (394.2266, 297.4729)
  line L372 (394.9766, 298.7719) -> (383.1914, 319.1845)
  line L373 (381.6914, 319.1845) -> (377.3664, 311.6934)
  line L374 (377.3664, 311.6934) -> (374.6817, 313.2434)
  line L375 (374.6817, 313.2434) -> (379.0067, 320.7345)
  line L376 (378.2567, 322.0335) -> (354.6863, 322.0335)
  line L377 (353.9363, 320.7345) -> (358.2613, 313.2434)
  line L378 (358.2613, 313.2434) -> (355.5766, 311.6934)
  line L379 (355.5766, 311.6934) -> (351.2516, 319.1845)
  line L380 (349.7516, 319.1845) -> (337.9664, 298.7719)
  line L381 (338.7164, 297.4729) -> (347.3664, 297.4729)
  line L382 (347.3664, 297.4729) -> (347.3664, 294.3729)
  line L383 (347.3664, 294.3729) -> (338.7164, 294.3729)
  line L384 (337.9663, 130.4099) -> (349.7515, 109.9973)
  line L385 (351.2515, 109.9973) -> (355.5765, 117.4884)
  line L386 (355.5765, 117.4884) -> (358.2612, 115.9384)
  line L387 (358.2612, 115.9384) -> (353.9362, 108.4473)
  line L388 (354.6862, 107.1482) -> (378.2566, 107.1482)